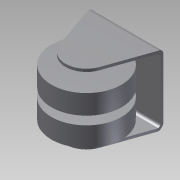
# Autodesk Inventor part: wheel
Saved by Autodesk Inventor 2012 (Build 160160000, 160)
## iProperties
Created: 2012-04-18
Part Number: wheel
Material: Default
Document SubType Name: Sheet Metal
Designer: thanos
Density: 1 g/cm^3
Sheet Metal Rule: Default_mm
Mass: 64.668 g
Surface Area: 251.975 cm^2
Volume: 64.668 cm^3
Author: thanos
Autodesk Inventor part; units mm, degrees
ref_plane "YZ Plane" through (0, 0, 0) normal (1, 0, 0) x (0, 1, 0)
ref_plane "XZ Plane" through (0, 0, 0) normal (0, 1, 0) x (-1, 0, 0)
ref_plane "XY Plane" through (0, 0, 0) normal (0, 0, 1) x (1, 0, 0)
sketch "Sketch3" plane through (0, 0, 0) normal (0, 0, 1) x (1, 0, 0)
  line L0 (-14.3279, -4.4399) -> (-25, 30)
  line L1 (-25, 30) -> (25, 30)
  line L2 (25, 30) -> (14.3279, -4.4399)
  circle A0 centre (0, 0) radius 15
  line L3 (-25, 30) -> (25, 30)
  line L4 (25, 30) -> (25, -15)
  line L5 (25, -15) -> (-25, -15)
  line L6 (-25, -15) -> (-25, 30)
  dimension "d0" = 50
  dimension "d1" = 30
  dimension "d2" = 30
  dimension "d24" = 50
  measures "d0" distance of L0.end L1.end
  measures "d1" distance from line of L1 A0.centre
  measures "d2" diameter of A0
  measures "d24" distance between parallel lines of L6 L4
extrude "Plate1" add sketch "Sketch3" along normal blind 2
sketch "Sketch8" plane through (25, 28, 2) normal (0, 1, 0) x (-1, 0, 0)
  line L0 (50, 0) -> (0, 0)
  line L1 (0, 0) -> (0, -50)
  line L2 (0, -50) -> (50, -50)
  line L3 (50, -50) -> (50, 0)
  constraints: 4 end point, 4 other
edge flange "Flange3" height 50 angle 90 thickness 2 bend radius 2 thickness toward (0, 1, 0) relief tear relief width 2 relief depth 1 edges at (0, 30, 0) wall of the first edge with corners at (-25, 28, 2) (25, 28, 2) (25, 28, -48) (-25, 28, -48)
bend "Bend5"
corner "Corner3"
sketch "Sketch9" plane through (25, 30, -46) normal (0, 0, -1) x (-1, 0, 0)
  line L0 (50, 0) -> (0, 0)
  line L1 (0, 0) -> (0, -45)
  line L2 (0, -45) -> (50, -45)
  line L3 (50, -45) -> (50, 0)
  constraints: 4 end point, 4 other
edge flange "Flange4" height 45 angle 90 thickness 2 bend radius 2 thickness toward (0, 0, -1) relief tear relief width 2 relief depth 1 edges at (0, 28, -48) wall of the first edge with corners at (-25, 30, -46) (25, 30, -46) (25, -15, -46) (-25, -15, -46)
bend "Bend6"
corner "Corner4"
sketch "Sketch11" plane through (0, 0, 2) normal (0, 0, 1) x (1, 0, 0)
  line L0 (25, 26) -> (-25, 26) projected
  line L1 (-25, -15) -> (-25, 26) projected
  line L2 (25, -15) -> (-25, -15) projected
  line L3 (25, 26) -> (25, -15) projected
  arc A0 (-14.1568, -4.9584) -> (14.1568, -4.9584) centre (0, 0) ccw
  line L4 (-25, 26) -> (-14.1568, -4.9584)
  line L5 (25, 26) -> (14.1568, -4.9584)
  constraints: 4 end point, 3 tangent, 2 point on circle, 1 centre point, 1 coincident
extrude "Cut2" cut sketch "Sketch11" against normal through all contours L3 L2 A0 L5 | L4 A0 L2 L1
sketch "Sketch12" plane through (-25, 26, -46) normal (0, 0, 1) x (1, 0, 0)
  arc A0 (10.8432, -30.9584) -> (39.1568, -30.9584) centre (25, -26) ccw projected
  circle A1 centre (25, -26) radius 6
  dimension "d59" = 12
  constraints: 1 centre point, 1 coincident
  measures "d59" diameter of A1
extrude "Extrusion1" add sketch "Sketch12" along normal blind 6
sketch "Sketch13" plane through (0, 0, -40) normal (0, 0, 1) x (1, 0, 0)
  circle A0 centre (0, 0) radius 6 projected
  circle A1 centre (0, 0) radius 25
  dimension "d62" = 50
  constraints: 1 centre point, 1 coincident
  measures "d62" diameter of A1
extrude "Extrusion2" add sketch "Sketch13" along normal blind 14
sketch "Sketch14" plane through (0, 0, -26) normal (0, 0, 1) x (1, 0, 0)
  circle A0 centre (0, 0) radius 6 projected
extrude "Extrusion3" add sketch "Sketch14" along normal blind 6
sketch "Sketch15" plane through (0, 0, -20) normal (0, 0, 1) x (1, 0, 0)
  circle A0 centre (0, 0) radius 6 projected
  circle A1 centre (0, 0) radius 6 projected
  circle A2 centre (0, 0) radius 25 projected
extrude "Extrusion4" add sketch "Sketch15" along normal blind 14
sketch "Sketch16" plane through (0, 0, -6) normal (0, 0, 1) x (1, 0, 0)
  circle A0 centre (0, 0) radius 6 projected
extrude "Extrusion5" add sketch "Sketch16" along normal up to next
equation "\"d57\" = Thickness"
equation "\"d35\" = BendReliefWidth"
equation "\"d36\" = BendReliefDepth"
equation "\"d37\" = MinimumRemnant"
equation "\"d38\" = BendRadius"
equation "\"d41\" = BendRadius"
equation "\"d42\" = CornerReliefSize"
equation "\"d43\" = GapSize"
equation "\"d44\" = JacobiRadiusSize"
equation "\"d45\" = BendReliefWidth"
equation "\"d46\" = BendReliefDepth"
equation "\"d47\" = MinimumRemnant"
equation "\"d48\" = BendRadius"
equation "\"d51\" = BendRadius"
equation "\"d52\" = CornerReliefSize"
equation "\"d53\" = GapSize"
equation "\"d54\" = JacobiRadiusSize"
equation "\"BendRadius\" = Thickness"
equation "\"BendReliefWidth\" = Thickness"
equation "\"BendReliefDepth\" = 0.5 * Thickness"
equation "\"CornerReliefSize\" = 4 * Thickness"
equation "\"MinimumRemnant\" = 2 * Thickness"
equation "\"TransitionRadius\" = BendRadius"
equation "\"JacobiRadiusSize\" = BendRadius"
equation "\"GapSize\" = Thickness"
equation "\"d3\" = BendRadius"
equation "\"Thickness\" = 2"
body "Solid1"
